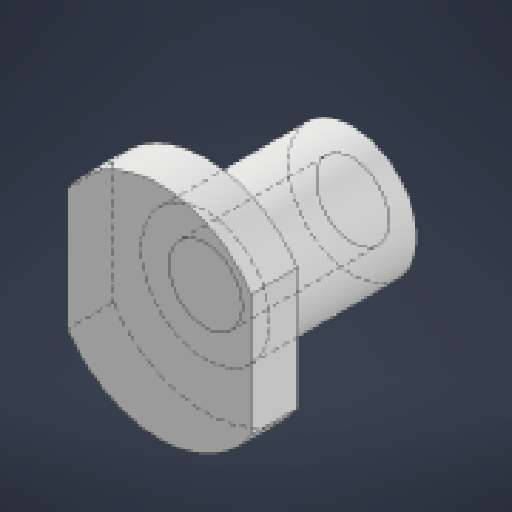
# Autodesk Inventor part: BALL_NUT
Saved by Autodesk Inventor 2023 (Build 270158000, 158)
## iProperties
Created: 2025-09-04
Part Number: BALL_NUT
Material: 일반
Document SubType Name: Modeling
Designer: k
Density: 1 g/cm^3
Appearance: 기본값
Author: k
Autodesk Inventor part; units mm, degrees
ref_plane "YZ Plane" through (0, 0, 0) normal (1, 0, 0) x (0, 1, 0)
ref_plane "XZ Plane" through (0, 0, 0) normal (0, 1, 0) x (-1, 0, 0)
ref_plane "XY Plane" through (0, 0, 0) normal (0, 0, 1) x (1, 0, 0)
sketch "스케치1" plane through (0, 0, 0) normal (0, 0, 1) x (1, 0, 0)
  circle A0 centre (-27.899, 28.5221) radius 24
  line L0 (-47.899, 60.3293) -> (-47.899, -6.0933)
  line L1 (-7.899, 60.3293) -> (-7.899, -6.0933)
  point P0 (0, 0)
  point P1 (-7.899, 15.2556)
  point P2 (-7.899, 41.7886)
  point P3 (-47.899, 41.7886)
  point P4 (-47.899, 15.2556)
  dimension "d0" = 48
  dimension "d1" = 20
  dimension "d2" = 40
  constraints: 4 end point, 1 centre point, 1 parallel, 1 vertical
  measures "d0" diameter of A0
  measures "d1" distance from line of A0.centre L0
  measures "d2" distance between parallel lines of L0 L1
extrude "돌출1" add sketch "스케치1" along normal blind 10 contours L1 A0 L0
sketch "스케치2" plane through (0, 0, 0) normal (0, 0, -1) x (-1, 0, 0)
  arc A0 (47.899, 41.7886) -> (7.899, 41.7886) centre (27.899, 28.5221) ccw projected
  circle A1 centre (27.899, 28.5221) radius 14
  point P0 (0, 0)
  dimension "d5" = 28
  constraints: 1 centre point, 1 coincident
  measures "d5" diameter of A1
extrude "돌출2" add sketch "스케치2" along normal blind 32
sketch "스케치3" plane through (-27.899, 28.5221, -32) normal (0, 0, -1) x (-1, 0, 0)
  circle A0 centre (0, 0) radius 14 projected
  circle A1 centre (0, 0) radius 8
  point P0 (-27.899, -28.5221)
  dimension "d8" = 16
  constraints: 1 centre point, 1 coincident
  measures "d8" diameter of A1
extrude "돌출3" cut sketch "스케치3" against normal through all contours A1
thread "스레드1" size "TR16x4" class "7H" standard "ISO Metric Trapezoidal Threads" full length
sketch "스케치4" plane through (0, 0, 10) normal (0, 0, 1) x (1, 0, 0)
  circle A0 centre (-27.899, 28.5221) radius 8 projected
  circle A1 centre (-27.899, 28.5221) radius 19
  circle A2 centre (-27.899, 9.5221) radius 2.75
  line L0 (-27.899, 28.5221) -> (-50.1984, 6.2227)
  line L1 (-27.899, 28.5221) -> (3.6371, 28.5221) construction
  line L2 (-27.899, 28.5221) -> (-27.899, -8.8486)
  circle A3 centre (-41.334, 15.087) radius 2.75
  circle A4 centre (-14.464, 15.087) radius 2.75
  circle A5 centre (-27.899, 47.5221) radius 2.75
  circle A6 centre (-41.334, 41.9571) radius 2.75
  circle A7 centre (-14.464, 41.9571) radius 2.75
  point P0 (0, 0)
  dimension "d15" = 38
  dimension "d16" = 5.5
  dimension "d17" = 135
  dimension "d18" = 5.5
  constraints: 7 centre point, 6 end point, 4 symmetric about line, 2 point on circle, 1 coincident, 1 equal length, 1 horizontal, 1 point on line, 1 vertical, 4 other
  measures "d15" diameter of A1
  measures "d16" diameter of A2
  measures "d17" angle of L0 L1
  measures "d18" diameter of A3
extrude "돌출4" cut sketch "스케치4" against normal blind 10 contours A3 A1 L0 | L0 A1 A3 | L2 A1 A2 | A2 A1 L2 | L0 A3 A1 | A1 A3 L0 | A2 L2 A1 | A1 L2 A2 | A6 A1 | A1 A6 | A4 A1 | A1 A4 | A5 A1 | A1 A5 | A7 A1 | A1 A7
